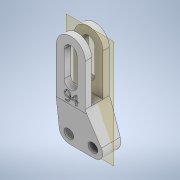
# Autodesk Inventor part: 1번부품
Saved by Autodesk Inventor 2022 (Build 260153000, 153)
## iProperties
Created: 2021-09-05
Part Number: 1번부품
Material: 일반
Document SubType Name: Modeling
Designer: 서울공업고등학교
Density: 1 g/cm^3
Appearance: 기본값
Author: 서울공업고등학교
Autodesk Inventor part; units mm, degrees
ref_plane "YZ Plane" through (0, 0, 0) normal (1, 0, 0) x (0, 1, 0)
ref_plane "XZ Plane" through (0, 0, 0) normal (0, 1, 0) x (-1, 0, 0)
ref_plane "XY Plane" through (0, 0, 0) normal (0, 0, 1) x (1, 0, 0)
sketch "스케치1" plane through (0, 0, 0) normal (0, 0, 1) x (1, 0, 0)
  line L0 (0, 0) -> (18, 0)
  line L1 (18, 26) -> (18, 61)
  line L2 (18, 61) -> (0, 61)
  line L3 (0, 61) -> (0, 0)
  line L4 (0, 26) -> (18, 26)
  line L5 (0, 0) -> (27, 0)
  circle A0 centre (6, 6) radius 3
  circle A1 centre (21, 6) radius 3
  arc A2 (21, 0) -> (26.4024, 8.6104) centre (21, 6) ccw
  line L6 (18, 26) -> (26.4024, 8.6104)
  line L7 (9, 52) -> (9, 36) construction
  line L8 (5, 52) -> (5, 36)
  line L9 (13, 36) -> (13, 52)
  arc A3 (13, 52) -> (5, 52) centre (9, 52) ccw
  arc A4 (5, 36) -> (13, 36) centre (9, 36) ccw
  point P0 (9, 44)
  dimension "d0" = 18
  dimension "d1" = 61
  dimension "d2" = 35
  dimension "d3" = 27
  dimension "d4" = 6
  dimension "d5" = 6
  dimension "d6" = 6
  dimension "d7" = 6
  dimension "d8" = 15
  dimension "d9" = 12
  dimension "d11" = 16
  dimension "d13" = 4
  dimension "d14" = 9
  dimension "d15" = 52
  constraints: 22 end point, 6 point on circle, 5 centre point, 5 tangent, 4 parallel, 3 point on line, 2 perpendicular, 1 coincident, 1 horizontal, 1 horizontal alignment, 1 midpoint
  measures "d0" distance of L1.end L2.end
  measures "d1" distance of L2.end L0.start
  measures "d2" distance between parallel lines of L4 L2
  measures "d3" distance of L0.start L5.end
  measures "d4" diameter of A0
  measures "d5" diameter of A1
  measures "d6" distance from line of L0 A0.centre
  measures "d7" distance from line of L3 A0.centre
  measures "d8" distance of A1.centre A0.centre
  measures "d9" diameter of A2
  measures "d11" distance of L7.end L7.start
  measures "d13" radius of A3
  measures "d14" distance from line of L3 point (9, 44)
  measures "d15" distance from line of L0 L7.start
extrude "돌출1" add sketch "스케치1" along normal mid plane 15
fillet "모깎기1" radius 9 2 edges at (18, 61, 0) (0, 61, 0)
fillet "모깎기2" radius 6 1 edges at (0, 0, 0)
sketch "스케치2" plane through (0, 52, -7.5) normal (-1, 0, 0) x (0, 0, 1)
  line L0 (0, -52) -> (15, -52) projected
  line L1 (0, -43.3896) -> (0, -52) projected
  line L2 (0, -52) -> (2.5225, -52)
  line L3 (0, -26) -> (0, -43.3896) projected
  line L4 (0, -28) -> (0, -52)
  line L5 (0, -28) -> (2.5225, -52)
  line L6 (15, -46) -> (0, -46) projected
  line L7 (15, 0) -> (15, -46) projected
  line L8 (0, 0) -> (15, 0) projected
  line L9 (0, -46) -> (0, 0) projected
  point P0 (7.5, -52)
  dimension "d20" = 24
  dimension "d21" = 6
  constraints: 6 end point, 2 point on line, 1 collinear
  measures "d20" distance from line of L0 L4.start
  measures "d21" angle of L1 L5
extrude "돌출2" cut sketch "스케치2" against normal through all contours L1 L6 L5 L0 | L1 L3 L5 L6
mirror "미러1" about plane through (0, 0, 0) normal (0, 0, 1) of "돌출2"
sketch "스케치3" plane through (0, 0, 7.5) normal (0, 0, 1) x (1, 0, 0)
  line L0 (4.9184, 31.221) -> (13.9232, 31.221) construction
  line L1 (13.9232, 31.221) -> (13.9232, 25.4105) construction
  line L2 (13.9232, 25.4105) -> (4.9184, 25.4105) construction
  line L3 (4.9184, 25.4105) -> (4.9184, 31.221) construction
  spline S0 degree 2 poles (5.1907, 29.1497) (5.1907, 29.6116) (5.4921, 30.3799) (5.7547, 30.657) knots 0 0 0 1 2 2 2
  spline S1 degree 2 poles (5.7547, 30.657) (6.0027, 30.9244) (6.7271, 31.221) (7.0967, 31.221) knots 0 0 0 1 2 2 2
  spline S2 degree 2 poles (7.0967, 31.221) (7.51, 31.221) (8.1809, 30.9439) (8.4289, 30.6813) knots 0 0 0 1 2 2 2
  spline S3 degree 2 poles (8.4289, 30.6813) (8.7401, 30.3507) (9.0805, 29.281) (9.0805, 28.4593) knots 0 0 0 1 2 2 2
  spline S4 degree 2 poles (9.0805, 28.4593) (9.0805, 27.7154) (8.745, 26.3831) (8.4192, 25.9406) knots 0 0 0 1 2 2 2
  spline S5 degree 2 poles (8.4192, 25.9406) (8.074, 25.4739) (7.1015, 24.9828) (6.3916, 24.9828) knots 0 0 0 1 2 2 2
  spline S6 degree 2 poles (6.3916, 24.9828) (6.2312, 24.9828) (5.8665, 25.0168) (5.7109, 25.0654) knots 0 0 0 1 2 2 2
  line L4 (5.7109, 25.0654) -> (5.7109, 25.8385)
  line L5 (5.7109, 25.8385) -> (5.7498, 25.8385)
  spline S7 degree 2 poles (5.7498, 25.8385) (5.8519, 25.7802) (6.2798, 25.6781) (6.4986, 25.6781) knots 0 0 0 1 2 2 2
  spline S8 degree 2 poles (6.4986, 25.6781) (7.2863, 25.6781) (8.1858, 26.7186) (8.249, 27.6813) knots 0 0 0 1 2 2 2
  spline S9 degree 2 poles (8.249, 27.6813) (7.9281, 27.4625) (7.3446, 27.2632) (6.9994, 27.2632) knots 0 0 0 1 2 2 2
  spline S10 degree 2 poles (6.9994, 27.2632) (6.6688, 27.2632) (6.1194, 27.409) (5.8422, 27.6181) knots 0 0 0 1 2 2 2
  spline S11 degree 2 poles (5.8422, 27.6181) (5.5213, 27.8661) (5.1907, 28.6197) (5.1907, 29.1497) knots 0 0 0 1 2 2 2
  spline S12 degree 2 poles (8.2685, 28.6392) (8.2685, 29.247) (8.0448, 30.0152) (7.8454, 30.2243) knots 0 0 0 1 2 2 2
  spline S13 degree 2 poles (7.8454, 30.2243) (7.6704, 30.4188) (7.3057, 30.5646) (7.0918, 30.5646) knots 0 0 0 1 2 2 2
  spline S14 degree 2 poles (7.0918, 30.5646) (6.5959, 30.5646) (6.0075, 29.8547) (6.0075, 29.1838) knots 0 0 0 1 2 2 2
  spline S15 degree 2 poles (6.0075, 29.1838) (6.0075, 28.8045) (6.202, 28.3134) (6.4159, 28.1384) knots 0 0 0 1 2 2 2
  spline S16 degree 2 poles (6.4159, 28.1384) (6.5715, 28.012) (6.9557, 27.9293) (7.1793, 27.9293) knots 0 0 0 1 2 2 2
  spline S17 degree 2 poles (7.1793, 27.9293) (7.437, 27.9293) (8.0302, 28.1092) (8.2539, 28.2599) knots 0 0 0 1 2 2 2
  spline S18 degree 2 poles (8.2539, 28.2599) (8.2587, 28.3183) (8.2685, 28.5176) (8.2685, 28.6392) knots 0 0 0 1 2 2 2
  line L6 (13.719, 27.1611) -> (13.0043, 27.1611)
  line L7 (13.0043, 27.1611) -> (13.0043, 25.0995)
  line L8 (13.0043, 25.0995) -> (12.2312, 25.0995)
  line L9 (12.2312, 25.0995) -> (12.2312, 27.1611)
  line L10 (12.2312, 27.1611) -> (9.5813, 27.1611)
  line L11 (9.5813, 27.1611) -> (9.5813, 28.0071)
  line L12 (9.5813, 28.0071) -> (12.2652, 31.0995)
  line L13 (12.2652, 31.0995) -> (13.0043, 31.0995)
  line L14 (13.0043, 31.0995) -> (13.0043, 27.8077)
  line L15 (13.0043, 27.8077) -> (13.719, 27.8077)
  line L16 (13.719, 27.8077) -> (13.719, 27.1611)
  line L17 (12.2312, 27.8077) -> (12.2312, 30.1513)
  line L18 (12.2312, 30.1513) -> (10.2134, 27.8077)
  line L19 (10.2134, 27.8077) -> (12.2312, 27.8077)
  point P0 (0, 0)
  constraints: 2 other
extrude "돌출3" cut sketch "스케치3" against normal blind 1
ref_plane "작업 평면1" through (0, 0, 0) normal (0, 0, 1) x (1, 0, 0)
sketch "스케치4" plane through (0, 0, 0) normal (0, 0, 1) x (1, 0, 0)
  line L0 (24.8661, 65.9707) -> (-7.4953, 65.9707)
  line L1 (-7.4953, 65.9707) -> (-7.4953, 26)
  line L2 (-7.4953, 26) -> (24.8661, 26)
  line L3 (24.8661, 26) -> (24.8661, 65.9707)
  point P0 (0, 0)
  dimension "d26" = 26
  constraints: 8 end point, 2 parallel, 1 horizontal, 1 perpendicular
  measures "d26" distance from line of point (0, 0) L2
extrude "돌출4" cut sketch "스케치4" along normal mid plane 7
